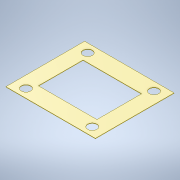
# Autodesk Inventor part: Part6
Saved by Autodesk Inventor 2020 (Build 240168000, 168)
## iProperties
Created: 2021-10-14
Part Number: Part6
Material: Nylon 6/6
Document SubType Name: Modeling
Designer: simon.erikssonwestl
Density: 1.13 g/cm^3
Appearance: Nylon 6
Author: simon.erikssonwestl
Autodesk Inventor part; units mm, degrees
ref_plane "YZ Plane" through (0, 0, 0) normal (1, 0, 0) x (0, 1, 0)
ref_plane "XZ Plane" through (0, 0, 0) normal (0, 1, 0) x (-1, 0, 0)
ref_plane "XY Plane" through (0, 0, 0) normal (0, 0, 1) x (1, 0, 0)
sketch "Sketch1" plane through (0, 0, 0) normal (0, 1, 0) x (-1, 0, 0)
  line L0 (14.5, 12.75) -> (-14.5, 12.75)
  line L1 (-14.5, 12.75) -> (-14.5, -12.75)
  line L2 (-14.5, -12.75) -> (14.5, -12.75)
  line L3 (14.5, -12.75) -> (14.5, 12.75)
  line L4 (14.5, 12.75) -> (-14.5, -12.75) construction
  line L5 (-14.5, 12.75) -> (14.5, -12.75) construction
  point P0 (0, 0)
  dimension "d0" = 29
  dimension "d1" = 25.5
  constraints: 12 end point, 2 midpoint, 2 parallel, 1 horizontal, 1 perpendicular
  measures "d0" distance of L2.end L1.end
  measures "d1" distance of L1.end L0.end
extrude "Extrusion1" add sketch "Sketch1" along normal mid plane 0.13
sketch "Sketch2" plane through (0, 0.065, 0) normal (0, 1, 0) x (1, 0, 0)
  circle A0 centre (-10.75, 10) radius 1.5
  line L0 (14.5, 12.75) -> (-14.5, 12.75) projected
  line L1 (-14.5, 12.75) -> (-14.5, -12.75) projected
  circle A1 centre (10.75, 10) radius 1.5
  circle A2 centre (-10.75, -10) radius 1.5
  circle A3 centre (10.75, -10) radius 1.5
  point P0 (0, 0)
  dimension "d4" = 3
  dimension "d5" = 2.75
  dimension "d6" = 3.75
  dimension "d9" = 21.5
  dimension "d12" = 20
  constraints: 4 centre point, 1 horizontal, 1 vertical, 6 other
  measures "d4" diameter of A0
  measures "d5" distance from line of L0 A0.centre
  measures "d6" distance from line of L1 A0.centre
  measures "d9" distance of A0.centre A1.centre
  measures "d12" distance of A0.centre A2.centre
extrude "Extrusion2" cut sketch "Sketch2" against normal through all
sketch "Sketch3" plane through (0, 0.065, 0) normal (0, 1, 0) x (1, 0, 0)
  line L0 (-9.5, 7.25) -> (9.5, 7.25)
  line L1 (9.5, 7.25) -> (9.5, -7.25)
  line L2 (9.5, -7.25) -> (-9.5, -7.25)
  line L3 (-9.5, -7.25) -> (-9.5, 7.25)
  line L4 (-9.5, 7.25) -> (9.5, -7.25) construction
  line L5 (9.5, 7.25) -> (-9.5, -7.25) construction
  point P0 (0, 0)
  dimension "d17" = 19
  dimension "d18" = 14.5
  constraints: 12 end point, 2 midpoint, 2 parallel, 1 horizontal, 1 perpendicular
  measures "d17" distance of L1.end L2.end
  measures "d18" distance of L0.end L1.end
extrude "Extrusion3" cut sketch "Sketch3" against normal through all
body "Solid1"
